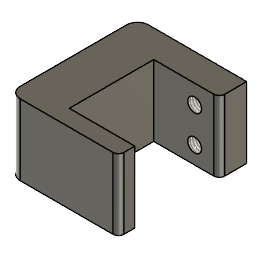
deck2bedClamp_I1 (Autodesk Fusion 360 design; units mm, degrees)
part number: 2026-05-03-05-26-52-082
Autodesk Fusion 360 part; units mm, degrees
sketch "Sketch1" plane through (0, 0, 0) normal (0, 1, 0) x (1, 0, 0)
  line L0 (-6.9583, -4.2531) -> (13.0417, -4.2531)
  line L1 (13.0417, -4.2531) -> (13.0417, 8.7469)
  line L2 (13.0417, 8.7469) -> (-6.9583, 8.7469)
  line L3 (-6.9583, 8.7469) -> (-6.9583, -4.2531)
  line L4 (-6.9583, -4.2531) -> (1.0417, -4.2531)
  line L5 (1.0417, -4.2531) -> (1.0417, 8.7469)
  line L6 (1.0417, 8.7469) -> (-6.9583, 8.7469)
  line L7 (-6.9583, 8.7469) -> (-6.9583, -4.2531)
  dimension "d4" = 20
  dimension "d5" = 13
  dimension "d7" = 8
  dimension "d8" = 13
  constraint horizontal L0
  constraint vertical L1
  constraint horizontal L2
  constraint vertical L3
  constraint horizontal L4
  constraint vertical L5
  constraint horizontal L6
  constraint vertical L7
  measures "d4" distance of L0.start L0.end
  measures "d5" distance of L0.start L2.end
  measures "d7" distance of L0.start L4.end
  measures "d8" distance of L0.start L2.end
extrude "Extrude1" add sketch "Sketch1" along normal blind 23.5 contours L0 L2 L3 L4 L5 L6 L7
extrude "Extrude2" add sketch "Sketch1" along normal blind 3 contours L0 L1 L2 L5
sketch "Sketch2" plane through (1.0417, 0, 0) normal (1, 0, 0) x (0, 1, 0)
  line L0 (3, -8.7469) -> (23.5, -8.7469)
  line L1 (23.5, -8.7469) -> (23.5, 4.2531)
  line L2 (23.5, 4.2531) -> (3, 4.2531)
  line L3 (3, -0.2469) -> (18.5, -0.2469)
  line L4 (23.5, 4.2531) -> (18.4635, 4.2531)
  line L5 (18.4635, 4.2531) -> (18.4635, -8.7469)
  line L6 (18.4635, -8.7469) -> (23.5, -8.7469)
  line L7 (23.5, -8.7469) -> (23.5, 4.2531)
  line L8 (3, 4.2531) -> (3, -8.7469)
  dimension "d16" = 15.5
  constraint horizontal L4
  constraint vertical L5
  constraint horizontal L6
  constraint vertical L7
  constraint coincident L0 L5.end
  constraint coincident L1.end L2.start
  measures "d16" distance of L3.start L3.end
extrude "Extrude3" add sketch "Sketch2" along normal blind 12 contours L0 L1 L2 L4 L5 L6 L7
fillet "Fillet1" radius 2 1 edges at (-6.9583, 23.5, -2.2469)
fillet "Fillet2" radius 2 1 edges at (-6.9583, 0, -2.2469)
fillet "Fillet3" radius 1 1 edges at (13.0417, 18.4635, -2.2469)
fillet "Fillet4" radius 1 1 edges at (13.0417, 0, -2.2469)
sketch "Sketch3" plane through (0, 23.5, 0) normal (0, 1, 0) x (-1, 0, 0)
  line L0 (4.9583, -8.7469) -> (4.9583, 4.2531)
  line L1 (4.9583, 4.2531) -> (-13.0417, 4.2531)
  line L2 (-13.0417, 4.2531) -> (-13.0417, -8.7469)
  line L3 (-13.0417, -8.7469) -> (4.9583, -8.7469)
  line L4 (4.9583, -2.2469) -> (-13.0417, -2.2469)
  line L5 (-8.5241, 4.0524) -> (-8.5241, 0.8024)
  line L6 (-8.5417, -8.8028) -> (-8.5417, -5.5528)
  circle A0 centre (-8.5241, 0.8024) radius 1.3
  circle A1 centre (-8.5417, -5.5528) radius 1.3
  line L7 (-13.0417, 0.8028) -> (-8.5417, 0.8028)
  line L8 (-13.0417, -5.5528) -> (-8.5417, -5.5528)
  dimension "d32" = 3.25
  dimension "d33" = 3.25
  dimension "d34" = 2.6
  dimension "d35" = 2.6
  dimension "d36" = 4.5
  dimension "d37" = 4.5
  constraint midpoint L0 L4.start
  constraint midpoint L2 L4.end
  constraint perpendicular L1 L5
  constraint perpendicular L3 L6
  constraint coincident L5.end A0.centre
  constraint coincident L6.end A1.centre
  constraint coincident L2 L7.start
  constraint perpendicular L2 L7
  constraint coincident L2 L8.start
  constraint perpendicular L2 L8
  measures "d32" distance of L5.start L5.end
  measures "d33" distance of L6.start L6.end
  measures "d34" diameter of A0
  measures "d35" diameter of A1
  measures "d36" distance of L7.start L7.end
  measures "d37" distance of L8.start L6.end
hole "Hole2" at (8.5417, 23.5, 0.8028) at (8.5417, 23.5, -5.5528) direction (0, -1, 0) diameter 2.529 depth 10 tip angle 118
thread "Thread2" "ISO Metric profile 3.0 M3x0.5 M3x0.5 6H" thread offset 0 thread depth 7.4
equation "clamp_w = 20 mm"
equation "clamp_l = 13 mm"
equation "clamp_bot_thickness = 3 mm"
equation "d4 = clamp_w"
equation "d5 = clamp_l"
equation "clamp_mid_w = 8 mm"
equation "d7 = clamp_mid_w"
equation "d8 = clamp_l"
equation "clamp_mid_thickness = deck_bed_gap + clamp_bot_thickness + clamp_top_thickness"
equation "d10 = clamp_mid_thickness"
equation "d12 = clamp_bot_thickness"
equation "clamp_top_thickness = 5 mm"
equation "deck_bed_gap = 15.5 mm"
equation "d16 = deck_bed_gap"
equation "top_clamp_depth = clamp_w - clamp_mid_w"
equation "d18 = top_clamp_depth"
